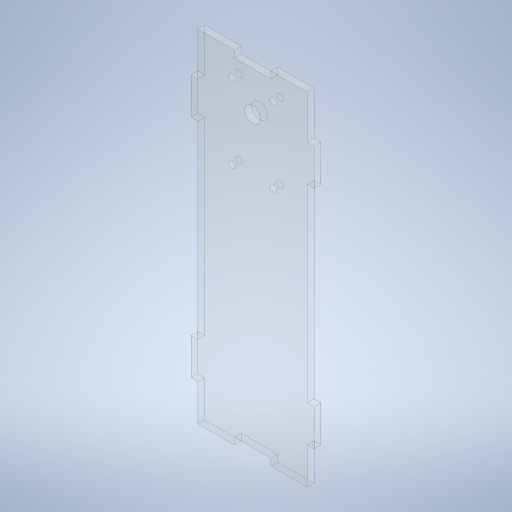
# Autodesk Inventor part: side plate
Saved by Autodesk Inventor 2023 (Build 270158000, 158)
## iProperties
Created: 2023-06-06
Part Number: side plate
Material: PMMA Plastic
Document SubType Name: Sheet Metal
Designer: Ronan
Density: 1.188 g/cm^3
Sheet Metal Rule: Default_mm
Appearance: Polycarbonate - Clear
Author: Ronan
Autodesk Inventor part; units mm, degrees
ref_plane "YZ Plane" through (0, 0, 0) normal (1, 0, 0) x (0, 1, 0)
ref_plane "XZ Plane" through (0, 0, 0) normal (0, 1, 0) x (-1, 0, 0)
ref_plane "XY Plane" through (0, 0, 0) normal (0, 0, 1) x (1, 0, 0)
sketch "Sketch1" plane through (0, 0, 0) normal (0, 0, 1) x (1, 0, 0)
  circle A0 centre (23, 103.0491) radius 1.5
  circle A1 centre (5, 103.0491) radius 1.5
  circle A2 centre (23, 136.0491) radius 1.5
  line L0 (-10, 144.0491) -> (38, 144.0491)
  line L1 (38, 144.0491) -> (38, -2.9509)
  line L2 (38, -2.9509) -> (-10, -2.9509)
  line L3 (-10, -2.9509) -> (-10, 144.0491)
  circle A3 centre (5, 136.0491) radius 1.5
  circle A4 centre (14, 126.5491) radius 3.5
  point P0 (0, 0)
  point P1 (14, 22.75)
  dimension "d10" = 3
  dimension "d12" = 3
  dimension "d13" = 3
  dimension "d14" = 3
  dimension "d15" = 33
  dimension "d16" = 18
  dimension "d17" = 18
  dimension "d18" = 33
  dimension "d19" = 15
  dimension "d20" = 8
  dimension "d21" = 15
  dimension "d22" = 147
  dimension "d25" = 7
  dimension "d26" = 9.5
  dimension "d27" = 9
  dimension "d28" = 9
  dimension "d29" = 2.9509
  dimension "d30" = 10
  dimension "d31" = 0
  constraints: 8 end point, 5 centre point, 2 perpendicular, 1 horizontal, 1 vertical
  measures "d10" diameter of A2
  measures "d12" diameter of A3
  measures "d13" diameter of A1
  measures "d14" diameter of A0
  measures "d15" distance of A1.centre A3.centre
  measures "d16" distance of A2.centre A3.centre
  measures "d17" distance of A0.centre A1.centre
  measures "d18" distance of A0.centre A2.centre
  measures "d19" distance from line of L3 A1.centre
  measures "d20" distance from line of L0 A3.centre
  measures "d21" distance from line of L1 A0.centre
  measures "d22" distance between parallel lines of L2 L0
  measures "d25" diameter of A4
  measures "d26" vertical distance of A4.centre A2.centre
  measures "d27" horizontal distance of A4.centre A2.centre
  measures "d28" horizontal distance of A4.centre A3.centre
  measures "d29" distance from line of point (0, 0) L2
  measures "d30" distance from line of point (0, 0) L3
  measures "d31" horizontal distance of A1.centre A3.centre
extrude "Extrusion1" add sketch "Sketch1" along normal blind 3
sketch "Sketch2" plane through (0, 0, 3) normal (0, 0, 1) x (1, 0, 0)
  line L0 (-10, 144.0491) -> (-10, -2.9509) projected
  line L1 (38, -2.9509) -> (38, 144.0491) projected
  line L2 (-10, 128.0491) -> (-13, 128.0491)
  line L3 (-13, 128.0491) -> (-13, 112.0491)
  line L4 (-13, 112.0491) -> (-10, 112.0491)
  line L5 (-10, 112.0491) -> (-10, 128.0491)
  line L6 (38, 128.0491) -> (41, 128.0491)
  line L7 (41, 128.0491) -> (41, 112.0491)
  line L8 (41, 112.0491) -> (38, 112.0491)
  line L9 (38, 112.0491) -> (38, 128.0491)
  line L10 (-10, 29.0491) -> (-13, 29.0491)
  line L11 (-13, 29.0491) -> (-13, 13.0491)
  line L12 (-13, 13.0491) -> (-10, 13.0491)
  line L13 (-10, 13.0491) -> (-10, 29.0491)
  line L14 (38, 29.0491) -> (41, 29.0491)
  line L15 (41, 29.0491) -> (41, 13.0491)
  line L16 (41, 13.0491) -> (38, 13.0491)
  line L17 (38, 13.0491) -> (38, 29.0491)
  line L18 (-10, -2.9509) -> (38, -2.9509) projected
  line L19 (38, 144.0491) -> (-10, 144.0491) projected
  line L20 (6, 144.0491) -> (22, 144.0491)
  line L21 (22, 144.0491) -> (22, 147.0491)
  line L22 (22, 147.0491) -> (6, 147.0491)
  line L23 (6, 147.0491) -> (6, 144.0491)
  line L24 (6, 144.0491) -> (-10, 144.0491)
  line L25 (-10, 144.0491) -> (-10, 147.0491)
  line L26 (-10, 147.0491) -> (6, 147.0491)
  line L27 (6, 147.0491) -> (6, 144.0491)
  line L28 (22, 144.0491) -> (38, 144.0491)
  line L29 (38, 144.0491) -> (38, 147.0491)
  line L30 (38, 147.0491) -> (22, 147.0491)
  line L31 (22, 147.0491) -> (22, 144.0491)
  point P0 (0, 0)
  point P1 (-11.5, 13.0491)
  point P2 (-10, 112.0491)
  point P3 (38, 112.0491)
  point P4 (22, 147.0491)
  point P5 (22, 144.0491)
  point P6 (-10, 144.0491)
  point P7 (6, 147.0491)
  dimension "d36" = 3
  dimension "d37" = 3
  dimension "d39" = 16
  dimension "d40" = 16
  dimension "d41" = 16
  dimension "d42" = 0
  dimension "d50" = 16
  dimension "d51" = 16
  dimension "d52" = 3
  dimension "d53" = 3
  dimension "d56" = 16
  constraints: 56 end point, 14 parallel, 11 point on line, 7 horizontal, 7 perpendicular, 3 collinear, 1 midpoint
  measures "d36" distance between parallel lines of L5 L3
  measures "d37" distance between parallel lines of L1 L7
  measures "d39" distance of L2.end L3.end
  measures "d40" distance of L10.end L11.end
  measures "d41" distance from line of L18 point (-11.5, 13.049)
  measures "d42" distance between parallel lines of L10 L14
  measures "d50" distance between parallel lines of L0 L23
  measures "d51" distance between parallel lines of L1 L21
  measures "d52" distance between parallel lines of L19 L22
  measures "d53" distance of L24.end L25.end
  measures "d56" distance between parallel lines of L19 L2
extrude "Extrusion2" add sketch "Sketch2" against normal blind 3 contours L25 L26 L23 L19 | L0 L4 L3 L2 | L21 L30 L29 L19 | L0 L12 L11 L10 | L6 L7 L8 L1 | L14 L15 L16 L1
sketch "Sketch4" plane through (0, 0, 3) normal (0, 0, 1) x (1, 0, 0)
  line L0 (-10, -2.9509) -> (38, -2.9509) projected
  line L1 (6, -2.9509) -> (22, -2.9509)
  line L2 (22, -2.9509) -> (22, 0.0491)
  line L3 (22, 0.0491) -> (6, 0.0491)
  line L4 (6, 0.0491) -> (6, -2.9509)
  line L5 (22, 144.0491) -> (6, 144.0491) projected
  line L6 (6, 144.0491) -> (6, 147.0491) projected
  point P0 (0, 0)
  constraints: 8 end point, 2 equal length, 2 parallel, 1 collinear, 1 horizontal, 1 perpendicular, 1 point on line
extrude "Extrusion4" cut sketch "Sketch4" against normal blind 3
equation "\"BendRadius\" = Thickness"
equation "\"BendReliefWidth\" = Thickness"
equation "\"BendReliefDepth\" = 0.5 * Thickness"
equation "\"CornerReliefSize\" = 4 * Thickness"
equation "\"MinimumRemnant\" = 2 * Thickness"
equation "\"TransitionRadius\" = BendRadius"
equation "\"JacobiRadiusSize\" = BendRadius"
equation "\"GapSize\" = Thickness"
equation "\"Thickness\" = 0.5"
body "Solid1"
